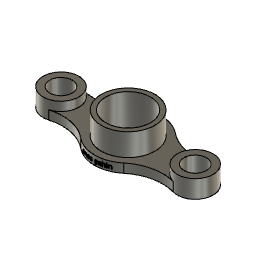
Model 28 (Autodesk Fusion 360 design; units mm, degrees)
Autodesk Fusion 360 part; units mm, degrees
sketch "Sketch1" plane through (0, 0, 0) normal (0, 0, 1) x (1, 0, 0)
  circle A0 centre (0, 0) radius 50
  circle A1 centre (0, 0) radius 60
  line L0 (0, 0) -> (150, 0) construction
  line L1 (0, 0) -> (-150, 0) construction
  circle A2 centre (150, 0) radius 25
  circle A3 centre (150, 0) radius 40
  circle A4 centre (-150, 0) radius 25
  circle A5 centre (-150, 0) radius 40
  arc A6 (-143.7829, 39.5139) -> (-48.0502, 57.5862) centre (-112.1172, 134.3679) ccw
  arc A7 (47.8929, 57.7172) -> (139.0714, 38.4781) centre (111.75, 134.6734) ccw
  arc A8 (139.0714, -38.4781) -> (47.8929, -57.7172) centre (111.75, -134.6734) ccw
  arc A9 (-47.8929, -57.7172) -> (-139.0714, -38.4781) centre (-111.75, -134.6734) ccw
  arc A10 (-47.8929, -57.7172) -> (47.8929, -57.7172) centre (0, 0) ccw
  arc A11 (47.8929, 57.7172) -> (-48.0502, 57.5862) centre (0, 0) ccw
  dimension "d1" = 100
  dimension "d2" = 120
  dimension "d3" = 150
  dimension "d4" = 150
  dimension "d5" = 150
  dimension "d6" = 50
  dimension "d7" = 80
  dimension "d8" = 50
  dimension "d9" = 80
  dimension "d10" = 200
  dimension "d11" = 200
  dimension "d12" = 200
  dimension "d13" = 200
  constraint coincident A0.centre A1.centre
  constraint concentric A0 A10
  constraint horizontal L0
  constraint parallel L0 L1
  constraint coincident L0.end A2.centre
  constraint coincident L1.end A4.centre
  constraint concentric A4 A5
  constraint tangent A6 A10
  constraint tangent A7 A10
  constraint tangent A3 A7
  constraint tangent A5 A9
  constraint tangent A9 A10
  constraint tangent A8 A10
  constraint tangent A3 A8
  constraint coincident A5 A6.start
  constraint coincident A3 A7.end
  constraint coincident A7.start A10
  constraint coincident A3 A8.start
  constraint coincident A5 A9.end
  constraint concentric A10 A11
  measures "d1" diameter of A0
  measures "d2" diameter of A1
  measures "d3" diameter of A10
  measures "d4" distance of A0.centre L0.end
  measures "d5" distance of A0.centre L1.end
  measures "d6" diameter of A2
  measures "d7" diameter of A3
  measures "d8" diameter of A4
  measures "d9" diameter of A5
  measures "d10" diameter of A6
  measures "d11" diameter of A7
  measures "d12" diameter of A8
  measures "d13" diameter of A9
extrude "Extrude1" add sketch "Sketch1" along normal blind 40 contours A3 | A5 A6 picked at (-147.2099, 34.8143) makes body 1 at (-147.6911, 39.9333, 26.6667) makes body 2 at (189.8012, -3.9827, 13.3333)
extrude "Extrude2" add sketch "Sketch1" along normal blind 70 separate body contours A1 makes body 3
extrude "Extrude3" add sketch "Sketch1" along normal blind 20 contours A3 A5 A6 A7 A8 A9 A10 A11 bodies 1 2 3
ref_plane "WorkPlane1" through (0, -75, 7.5055) normal (0, -1, 0) x (-1, 0, 0)
sketch "Sketch2" plane through (0, -75, 7.5055) normal (0, -1, 0) x (1, 0, 0)
  line L0 (-41.6787, 0) -> (40, 0) construction
  line L1 (40, 0) -> (40, 5.2952) construction
  line L2 (40, 5.2952) -> (-41.6787, 5.2952) construction
  line L3 (-41.6787, 5.2952) -> (-41.6787, 0) construction
  text T0 "enes şahin" font "Arial" height 10 align centre middle in box 81.6787 x 5.2952 at (-41.6787, 0) x (1, 0) y (0, 1) spacing 1
extrude "Extrude4" add sketch "Sketch2" along normal blind 0.5 from the near side of the face at (36.4781, -65.5313, 13.3333) text T0 on bodies 1 bodies 1
